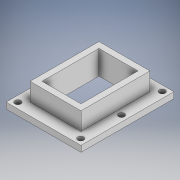
# Autodesk Inventor part: TipkaloDrzac_v.1.0
Saved by Autodesk Inventor 2020 (Build 240168000, 168)
## iProperties
Created: 2020-10-21
Part Number: TipkaloDrzac_v.1.0
Material: Generic
Document SubType Name: Modeling
Designer: Sičaja
Density: 1 g/cm^3
Appearance: Default
Author: Sičaja
Autodesk Inventor part; units mm, degrees
ref_plane "YZ Plane" through (0, 0, 0) normal (1, 0, 0) x (0, 1, 0)
ref_plane "XZ Plane" through (0, 0, 0) normal (0, 1, 0) x (-1, 0, 0)
ref_plane "XY Plane" through (0, 0, 0) normal (0, 0, 1) x (1, 0, 0)
sketch "Sketch1" plane through (0, 0, 0) normal (0, 1, 0) x (-1, 0, 0)
  line L0 (-6.5, -9.5) -> (6.5, -9.5)
  line L1 (6.5, -9.5) -> (6.5, 9.5)
  line L2 (6.5, 9.5) -> (-6.5, 9.5)
  line L3 (-6.5, 9.5) -> (-6.5, -9.5)
  line L4 (-6.5, -9.5) -> (6.5, 9.5) construction
  line L5 (6.5, -9.5) -> (-6.5, 9.5) construction
  line L6 (-8.5, -11.5) -> (8.5, -11.5)
  line L7 (8.5, -11.5) -> (8.5, 11.5)
  line L8 (8.5, 11.5) -> (-8.5, 11.5)
  line L9 (-8.5, 11.5) -> (-8.5, -11.5)
  line L10 (-8.5, -11.5) -> (8.5, 11.5) construction
  line L11 (8.5, -11.5) -> (-8.5, 11.5) construction
  point P0 (0, 0)
  dimension "d0" = 13
  dimension "d1" = 19
  dimension "d2" = 17
  dimension "d3" = 23
  constraints: 24 end point, 4 midpoint, 4 parallel, 2 horizontal, 2 perpendicular
  measures "d0" distance of L2.end L1.end
  measures "d1" distance of L1.end L0.end
  measures "d2" distance of L8.end L7.end
  measures "d3" distance of L7.end L6.end
extrude "Extrusion1" add sketch "Sketch1" along normal blind 8
sketch "Sketch2" plane through (0, 0, 0) normal (0, -1, 0) x (1, 0, 0)
  line L0 (8.5, 11.5) -> (8.5, -11.5) projected
  line L1 (-8.5, 11.5) -> (8.5, 11.5) projected
  line L2 (-8.5, -11.5) -> (-8.5, 11.5) projected
  line L3 (8.5, -11.5) -> (-8.5, -11.5) projected
  line L4 (-6.5, 9.5) -> (-6.5, -9.5) projected
  line L5 (6.5, 9.5) -> (-6.5, 9.5) projected
  line L6 (6.5, -9.5) -> (6.5, 9.5) projected
  line L7 (-6.5, -9.5) -> (6.5, -9.5) projected
  line L8 (-6.5, 9.5) -> (-6.5, -9.5) projected
  line L9 (6.5, 9.5) -> (-6.5, 9.5)
  line L10 (-6.5, 9.5) -> (-6.5, -9.5)
  line L11 (-6.5, -9.5) -> (6.5, -9.5)
  line L12 (6.5, -9.5) -> (6.5, 9.5)
  line L13 (6.5, 9.5) -> (-6.5, 9.5) projected
  line L14 (-6.5, -9.5) -> (6.5, -9.5) projected
  line L15 (6.5, -9.5) -> (6.5, 9.5) projected
  line L16 (6.5, 0) -> (12.5, 0)
  line L17 (12.5, 15.5) -> (-12.5, 15.5)
  line L18 (-12.5, 15.5) -> (-12.5, -15.5)
  line L19 (-12.5, -15.5) -> (12.5, -15.5)
  line L20 (12.5, -15.5) -> (12.5, 15.5)
  point P0 (0, 0)
  dimension "d9" = 25
  constraints: 18 end point, 4 parallel, 3 horizontal, 2 perpendicular, 1 midpoint
  measures "d9" distance of L19.end L18.end
extrude "Extrusion2" add sketch "Sketch2" against normal blind 2 contours L20 L19 L18 L17
sketch "Sketch3" plane through (0, 2, 0) normal (0, 1, 0) x (1, 0, 0)
  circle A0 centre (-10.4906, -13.5807) radius 1
  circle A1 centre (-10.5, 0) radius 1
  line L0 (-12.5, 15.5) -> (-12.5, -15.5) projected
  line L1 (-12.5, -15.5) -> (-12.5, 15.5)
  line L2 (-12.5, -15.5) -> (12.5, -15.5)
  circle A2 centre (-10.4906, 0.0193) radius 1
  circle A3 centre (-10.4906, 13.6193) radius 1
  line L3 (12.5, 15.5) -> (-12.5, 15.5) projected
  circle A4 centre (10.4906, -13.5807) radius 1
  circle A5 centre (10.4906, 0.0193) radius 1
  circle A6 centre (10.4906, 13.6193) radius 1
  point P0 (0, 0)
  point P1 (-11.3944, 0.4472)
  point P2 (-9.5962, -0.4279)
  dimension "d12" = 2
  dimension "d20" = 13.6
  constraints: 7 centre point, 4 end point, 2 vertical, 1 horizontal, 4 other
  measures "d12" diameter of A0
  measures "d20" distance of A0.centre A2.centre
extrude "Extrusion3" cut sketch "Sketch3" against normal blind 2 contours A0 | A1 A2 | A3 | A4 | A5 | A6 picked at (-10.303, 0.2798)
body "Solid1"
